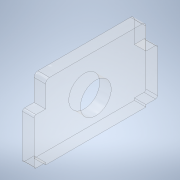
# Autodesk Inventor part: Laser-Pivot-Term-Beam
Saved by Autodesk Inventor 2021 (Build 250183000, 183)
## iProperties
Created: 2020-07-07
Part Number: Laser-Pivot-Term-Beam
Material: Acrylic, Clear
Document SubType Name: Modeling
Designer: lucas
Density: 1.19 g/cm^3
Appearance: Transparent - Clear
Project: 4Wire-Laser
Author: lucas
Revision Number: RLS_001
Autodesk Inventor part; units mm, degrees
ref_plane "YZ Plane" through (0, 0, 0) normal (1, 0, 0) x (0, 1, 0)
ref_plane "XZ Plane" through (0, 0, 0) normal (0, 1, 0) x (-1, 0, 0)
ref_plane "XY Plane" through (0, 0, 0) normal (0, 0, 1) x (1, 0, 0)
sketch "Sketch1" plane through (0, 0, 0) normal (1, 0, 0) x (0, 1, 0)
  circle A0 centre (0, 0) radius 4.05 construction
  line L0 (0, 0) -> (0, 16) construction
  line L1 (0, 0) -> (0, -16.0012) construction
  line L2 (1.45, -15.9997) -> (1.45, 0) construction
  line L3 (1.45, 0) -> (1.45, 16) construction
  line L4 (-7.75, -16) -> (-7.75, -9.5) construction
  line L5 (-7.75, 16) -> (-7.75, 9.5) construction
  line L6 (-2.8, -16.0023) -> (-2.8, 0) construction
  line L7 (-2.8, 0) -> (-2.8, 16) construction
  line L8 (-6, 16) -> (-6, 13)
  line L9 (-7.75, 9.5) -> (-7.75, -9.5) construction
  line L10 (-6.55, -11) -> (-7.75, -9.5) construction
  line L11 (-6.55, 11) -> (-7.75, 9.5) construction
  line L12 (5.5, 16) -> (-6, 16)
  line L13 (5.5, -16) -> (-4.55, -16)
  line L14 (-6, 16) -> (-7.75, 16) construction
  line L15 (-6, -13) -> (-6, -15.5)
  line L16 (-4.55, -16) -> (-6, -16)
  line L17 (-6, -13) -> (-6.55, -13)
  line L18 (-6.55, -13) -> (-6.55, -11.5)
  line L19 (-6.55, 11.5) -> (-6.55, 13)
  line L20 (-6.55, 13) -> (-6, 13)
  line L21 (-7.75, 9.5) -> (-6.55, 11) construction
  line L22 (-4.55, -16) -> (-5.5, -16) construction
  line L23 (-6, -16) -> (-7.75, -16) construction
  line L24 (6, -15.5) -> (6, -13)
  line L25 (6, 15.5) -> (6, 13)
  line L26 (12.6, 0) -> (-7.75, 0) construction
  line L27 (6, 13) -> (11.6, 13)
  line L28 (6, -13) -> (11.6, -13)
  circle A1 centre (1.45, 0) radius 4 construction
  line L29 (-6.05, 11) -> (-5.05, 11)
  line L30 (-4.55, 10.5) -> (-4.55, -10.5)
  line L31 (-5.05, -11) -> (-6.05, -11)
  arc A2 (-4.55, 10.5) -> (-5.05, 11) centre (-5.05, 10.5) ccw
  arc A3 (-5.05, -11) -> (-4.55, -10.5) centre (-5.05, -10.5) ccw
  arc A4 (-6.05, -11) -> (-6.55, -11.5) centre (-6.05, -11.5) ccw
  arc A5 (-6.55, 11.5) -> (-6.05, 11) centre (-6.05, 11.5) ccw
  line L32 (12.6, 12) -> (12.6, 0)
  line L33 (12.6, 0) -> (12.6, -12)
  line L34 (-6.55, 11.5) -> (-6.55, -11.5)
  line L35 (1.45, 0) -> (2, 0) construction
  circle A6 centre (2, 0) radius 4
  arc A7 (12.6, 12) -> (11.6, 13) centre (11.6, 12) ccw
  arc A8 (11.6, -13) -> (12.6, -12) centre (11.6, -12) ccw
  arc A9 (6, 15.5) -> (5.5, 16) centre (5.5, 15.5) ccw
  arc A10 (5.5, -16) -> (6, -15.5) centre (5.5, -15.5) ccw
  arc A11 (-6, -15.5) -> (-5.5, -16) centre (-5.5, -15.5) ccw
  point P0 (6, 16)
  point P1 (6, -16)
  point P2 (12.6, 13)
  point P3 (-6, -16)
  point P4 (12.6, -13)
  point P5 (-4.55, 11)
  dimension "d2" = 8.1
  dimension "d22" = 1.45
  dimension "d29" = 6.5
  dimension "d30" = 6.5
  dimension "d31" = 2.8
  dimension "d33" = 7.45
  dimension "d39" = 2
  dimension "d40" = 2
  dimension "d42" = 12
  dimension "d43" = 12
  dimension "d45" = 12
  dimension "d46" = 1.75
  dimension "d47" = 1.75
  dimension "d54" = 32
  dimension "d55" = 19
  dimension "d56" = 3
  dimension "d57" = 3
  dimension "d58" = 6.6
  dimension "d59" = 8
  dimension "d60" = 2
  dimension "d61" = 0.5
  dimension "d64" = 0.55
  dimension "d65" = 8
  dimension "d66" = 1
  dimension "d67" = 0.5
  constraints: 72 end point, 23 point on line, 18 point on circle, 18 tangent, 12 centre point, 12 perpendicular, 7 vertical, 6 equal radius, 6 horizontal, 3 coincident, 1 collinear, 1 midpoint, 2 other
  measures "d2" diameter of A0
  measures "d22" distance between parallel lines of L1 L2
  measures "d29" distance of L4.start L4.end
  measures "d30" distance of L5.start L5.end
  measures "d31" distance between parallel lines of L1 L6
  measures "d33" distance between parallel lines of L3 L8
  measures "d39" distance of L11.start L19.end
  measures "d40" distance of L17.end L10.start
  measures "d42" distance of L16.end point (6, -16)
  measures "d43" diameter of L15 L1
  measures "d45" diameter of L8 L0
  measures "d46" distance between parallel lines of L9 L8
  measures "d47" distance between parallel lines of L9 L15
  measures "d54" distance between parallel lines of L13 L12
  measures "d55" distance of L5.end L4.end
  measures "d56" distance of L8.start L8.end
  measures "d57" distance of L15.start L16.end
  measures "d58" distance of L25.end point (12.6, 13)
  measures "d59" diameter of A1
  measures "d60" distance of point (-6.55, 11) point (-4.55, 11)
  measures "d61" radius of A2
  measures "d64" distance of L35.start L35.end
  measures "d65" diameter of A6
  measures "d66" radius of A7
  measures "d67" radius of A9
extrude "Extrusion1" add sketch "Sketch1" along normal blind 3
fillet "Fillet1" radius 0.5 1 edges at (1.5, -6, 16)
body "Solid1"
